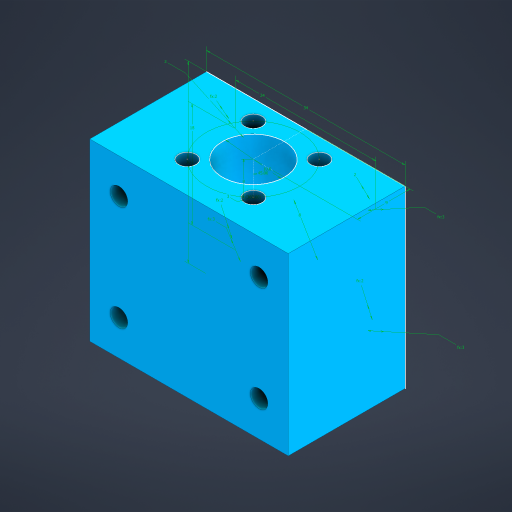
# Autodesk Inventor part: ZX Axis Carriage
Saved by Autodesk Inventor 2024.2 (Build 282272000, 272)
## iProperties
Created: 2024-10-02
Part Number: ZX Axis Carriage
Material: Generic
Document SubType Name: Modeling
Designer: jerem
Density: 1 g/cm^3
Appearance: Default
Author: jerem
Autodesk Inventor part; units mm, degrees
ref_plane "YZ Plane" through (0, 0, 0) normal (1, 0, 0) x (0, 1, 0)
ref_plane "XZ Plane" through (0, 0, 0) normal (0, 1, 0) x (-1, 0, 0)
ref_plane "XY Plane" through (0, 0, 0) normal (0, 0, 1) x (1, 0, 0)
sketch "Sketch1" plane through (0, 0, 0) normal (0, 0, 1) x (1, 0, 0)
  circle A0 centre (-12, 9) radius 1.5
  line L0 (12, -9) -> (-12, -9) construction
  line L1 (-12, -9) -> (-12, 9) construction
  line L2 (-12, 9) -> (12, 9) construction
  line L3 (12, 9) -> (12, -9) construction
  line L4 (12, -9) -> (-12, 9) construction
  line L5 (-12, -9) -> (12, 9) construction
  circle A1 centre (12, 9) radius 1.5
  circle A2 centre (12, -9) radius 1.5
  circle A3 centre (-12, -9) radius 1.5
  line L6 (17, -15) -> (-17, -15)
  line L7 (-17, -15) -> (-17, 15)
  line L8 (-17, 15) -> (17, 15)
  line L9 (17, 15) -> (17, -15)
  line L10 (17, -15) -> (-17, 15) construction
  line L11 (-17, -15) -> (17, 15) construction
  circle A4 centre (0, 0) radius 4
  circle A5 centre (12, 9) radius 3.5
  circle A6 centre (-12, 9) radius 3.5
  circle A7 centre (-12, -9) radius 3.5
  circle A8 centre (12, -9) radius 3.5
  point P0 (0, 0)
  dimension "d0" = 3
  dimension "d1" = 24
  dimension "d2" = 18
  dimension "d3" = 3
  dimension "d4" = 3
  dimension "d5" = 3
  dimension "d6" = 34
  dimension "d7" = 30
  dimension "d8" = 8
  dimension "d15" = 2
  dimension "d16" = 2
  dimension "d17" = 2
  dimension "d18" = 2
  constraints: 24 end point, 9 centre point, 9 coincident, 4 midpoint, 4 parallel, 2 horizontal, 2 perpendicular
  measures "d0" diameter of A0
  measures "d1" distance of L4.end L3.start
  measures "d2" distance of L0.end L4.end
  measures "d3" diameter of A3
  measures "d4" diameter of A1
  measures "d5" diameter of A2
  measures "d6" distance of L7.end L8.end
  measures "d7" distance of L6.end L7.end
  measures "d8" diameter of A4
  measures "d15" radial gap between concentric circles of A5 A1
  measures "d16" radial gap between concentric circles of A6 A0
  measures "d17" radial gap between concentric circles of A7 A3
  measures "d18" radial gap between concentric circles of A8 A2
extrude "Extrusion1" add sketch "Sketch1" along normal blind 20 contours L6 L7 L8 L9 | A4
extrude "Extrusion3" add sketch "Sketch1" against normal blind 5 from surface at 20 contours A5 | A6 | A7 | A8
sketch "Sketch2" plane through (-17, 15, 0) normal (0, 1, 0) x (1, 0, 0)
  circle A0 centre (17, -9) radius 5.3
  line L0 (17, -9) -> (17, 0) construction
  line L1 (17, -9) -> (22.6569, -14.6569) construction
  line L2 (17, -9) -> (25, -9) construction
  circle A1 centre (22.6569, -14.6569) radius 1.5
  circle A2 centre (22.6569, -3.3431) radius 1.5
  circle A3 centre (11.3431, -3.3431) radius 1.5
  circle A4 centre (11.3431, -14.6569) radius 1.5
  dimension "d11" = 10.6
  dimension "d12" = 9
  dimension "d21" = 45
  dimension "d22" = 8
  dimension "d23" = 3
  dimension "d26" = 360
  constraints: 6 end point, 5 centre point, 1 coincident, 1 equal length, 1 horizontal, 1 vertical, 9 other
  measures "d11" diameter of A0
  measures "d12" distance of L0.start L0.end
  measures "d21" angle of L1 L2
  measures "d22" distance of L0.start L1.end
  measures "d23" diameter of A1
extrude "Extrusion2" cut sketch "Sketch2" against normal through all contours A0
extrude "Extrusion4" cut sketch "Sketch2" against normal blind 10 contours A1 | A2 | A3 | A4
equation "\"d3\" = d0"
equation "\"d4\" = d0"
equation "\"d5\" = d0"
equation "\"d16\" = d15"
equation "\"d17\" = d15"
equation "\"d18\" = d15"
body "Solid1"
